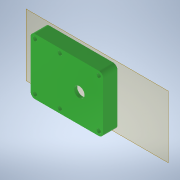
# Autodesk Inventor part: OutputFile
Saved by Autodesk Inventor 2022 (Build 260153000, 153)
## iProperties
Created: 2022-02-02
Part Number: OutputFile
Material: Generisch
Document SubType Name: Modeling
Designer: diederichbenedict
Density: 1 g/cm^3
Appearance: Glatt - Waldgrün
Mass: 24.3371 g
Surface Area: 140.293 cm^2
Volume: 24.3371 cm^3
Author: diederichbenedict
Autodesk Inventor part; units mm, degrees
ref_plane "YZ Plane" through (0, 0, 0) normal (1, 0, 0) x (0, 1, 0)
ref_plane "XZ Plane" through (0, 0, 0) normal (0, 1, 0) x (-1, 0, 0)
ref_plane "Arbeitsebene1" through (0, 0, 0) normal (0, 0, 1) x (1, 0, 0)
sketch "Skizze1" plane through (0, 0, 0) normal (0, 0, 1) x (1, 0, 0)
  arc A0 (-16.0148, -15.7672) -> (-14.255, -16.2126) centre (-14.255, -12.5126) ccw projected
  line L0 (-17.955, -12.5126) -> (-17.955, 12.4874) projected
  arc A1 (-14.255, 16.1874) -> (-17.955, 12.4874) centre (-14.255, 12.4874) ccw projected
  line L1 (-14.255, 16.1874) -> (23.745, 16.1874) projected
  arc A2 (25.6605, 15.6531) -> (23.745, 16.1874) centre (23.745, 12.4874) ccw projected
  arc A3 (26.3244, -15.1653) -> (27.445, -12.5126) centre (23.745, -12.5126) ccw projected
  line L2 (23.745, -16.2126) -> (-14.255, -16.2126) projected
  line L3 (-17.2153, 19.4874) -> (26.7847, 19.4874) projected
  arc A4 (-17.2153, 19.4874) -> (-20.2153, 16.4874) centre (-17.2153, 16.4874) ccw projected
  line L4 (-20.2153, -16.4874) -> (-20.2153, 16.4874) projected
  arc A5 (-20.2153, -16.4874) -> (-17.2153, -19.4874) centre (-17.2153, -16.4874) ccw projected
  line L5 (26.7847, -19.4874) -> (-17.2153, -19.4874) projected
  arc A6 (-16.0148, -15.7672) -> (-14.255, -16.2126) centre (-14.255, -12.5126) ccw projected
  line L6 (-17.955, -12.5126) -> (-17.955, 12.4874) projected
  arc A7 (-14.255, 16.1874) -> (-17.955, 12.4874) centre (-14.255, 12.4874) ccw projected
  line L7 (-14.255, 16.1874) -> (23.745, 16.1874) projected
  arc A8 (25.6605, 15.6531) -> (23.745, 16.1874) centre (23.745, 12.4874) ccw projected
  arc A9 (26.3244, -15.1653) -> (27.445, -12.5126) centre (23.745, -12.5126) ccw projected
  line L8 (23.745, -16.2126) -> (-14.255, -16.2126) projected
  line L9 (-17.2153, 19.4874) -> (26.7847, 19.4874) projected
  line L10 (26.7847, -19.4874) -> (-17.2153, -19.4874) projected
  line L11 (-20.2153, -16.4874) -> (-20.2153, 16.4874) projected
  arc A10 (-20.2153, -16.4874) -> (-17.2153, -19.4874) centre (-17.2153, -16.4874) ccw projected
  line L12 (29.7847, 16.4874) -> (29.7847, 15.1761) projected
  arc A11 (29.7847, 16.4874) -> (26.7847, 19.4874) centre (26.7847, 16.4874) ccw projected
  arc A12 (26.7847, -19.4874) -> (29.7847, -16.4874) centre (26.7847, -16.4874) ccw projected
  line L13 (29.7847, 16.4874) -> (29.7847, 15.1761) projected
  arc A13 (29.7847, 16.4874) -> (26.7847, 19.4874) centre (26.7847, 16.4874) ccw projected
  arc A14 (26.7847, -19.4874) -> (29.7847, -16.4874) centre (26.7847, -16.4874) ccw projected
  line L14 (28.445, 12.4874) -> (28.445, -12.5126)
  arc A15 (26.2819, 15.1808) -> (25.6605, 15.6531) centre (26.7847, 16.4874) ccw projected
  arc A16 (23.745, -16.2126) -> (25.6293, -15.6968) centre (23.745, -12.5126) ccw projected
  arc A17 (25.6293, -15.6968) -> (26.3244, -15.1653) centre (26.7847, -16.4874) ccw projected
  arc A18 (-16.8692, -15.1309) -> (-16.0148, -15.7672) centre (-17.2153, -16.4874) ccw projected
  arc A19 (27.3804, 13.1761) -> (26.2819, 15.1808) centre (23.745, 12.4874) ccw projected
  line L15 (23.745, 13.4874) -> (-14.255, 13.4874) projected
  line L16 (-14.255, -13.5126) -> (23.745, -13.5126) projected
  line L17 (25.0985, -12.5126) -> (27.445, -12.5126) projected
  arc A20 (-17.955, -12.5126) -> (-16.8692, -15.1309) centre (-14.255, -12.5126) ccw projected
  arc A21 (26.2819, 15.1808) -> (25.6605, 15.6531) centre (26.7847, 16.4874) ccw projected
  arc A22 (23.745, -16.2126) -> (25.6293, -15.6968) centre (23.745, -12.5126) ccw projected
  arc A23 (25.6293, -15.6968) -> (26.3244, -15.1653) centre (26.7847, -16.4874) ccw projected
  arc A24 (-16.8692, -15.1309) -> (-16.0148, -15.7672) centre (-17.2153, -16.4874) ccw projected
  arc A25 (27.3804, 13.1761) -> (26.2819, 15.1808) centre (23.745, 12.4874) ccw projected
  line L18 (23.745, 13.4874) -> (-14.255, 13.4874) projected
  line L19 (-14.255, -13.5126) -> (23.745, -13.5126) projected
  line L20 (25.0985, -12.5126) -> (27.445, -12.5126) projected
  arc A26 (-17.955, -12.5126) -> (-16.8692, -15.1309) centre (-14.255, -12.5126) ccw projected
  circle A27 centre (-17.2153, 16.4874) radius 1.15
  circle A28 centre (26.7847, 16.4874) radius 1.4
  circle A29 centre (26.7847, -16.4874) radius 1.4
  circle A30 centre (-17.2153, -16.4874) radius 1.4
  circle A31 centre (-17.2153, 16.4874) radius 1.15 projected
  circle A32 centre (-17.2153, 16.4874) radius 1.15 projected
  line L21 (25.0985, -9.7969) -> (25.0985, -12.5126) projected
  line L22 (18.0985, 10.1761) -> (-2.8285, 10.1761) projected
  line L23 (-2.8285, 10.1761) -> (-2.8285, 13.1761) projected
  arc A33 (24.4701, 13.1761) -> (23.745, 13.4874) centre (23.745, 12.4874) ccw projected
  arc A34 (23.745, -13.5126) -> (24.7038, -12.7969) centre (23.745, -12.5126) ccw projected
  line L24 (24.7038, -12.7969) -> (-2.8285, -12.7969) projected
  line L25 (-2.8285, -12.7969) -> (-2.8285, -9.7969) projected
  line L26 (-2.8285, -9.7969) -> (25.0985, -9.7969) projected
  circle A35 centre (-17.2153, 16.4874) radius 1.15 projected
  circle A36 centre (-17.2153, 16.4874) radius 1.15 projected
  line L27 (25.0985, -9.7969) -> (25.0985, -12.5126) projected
  line L28 (18.0985, 10.1761) -> (-2.8285, 10.1761) projected
  line L29 (-2.8285, 10.1761) -> (-2.8285, 13.1761) projected
  arc A37 (24.4701, 13.1761) -> (23.745, 13.4874) centre (23.745, 12.4874) ccw projected
  arc A38 (23.745, -13.5126) -> (24.7038, -12.7969) centre (23.745, -12.5126) ccw projected
  line L30 (24.7038, -12.7969) -> (-2.8285, -12.7969) projected
  line L31 (-2.8285, -12.7969) -> (-2.8285, -9.7969) projected
  line L32 (-2.8285, -9.7969) -> (25.0985, -9.7969) projected
  line L33 (27.445, 12.4874) -> (27.445, -12.5126)
  arc A39 (27.7847, 13.1761) -> (29.7847, 15.1761) centre (27.7847, 15.1761) ccw projected
  arc A40 (-17.2153, 19.4874) -> (-20.2153, 16.4874) centre (-17.2153, 16.4874) ccw projected
  line L34 (29.7847, 2.2345) -> (29.7847, -16.4874) projected
  arc A41 (29.7847, 2.2345) -> (27.7847, 4.2345) centre (27.7847, 2.2345) ccw projected
  line L35 (27.7847, 4.2345) -> (22.0985, 4.2345) projected
  arc A42 (20.0985, 6.2345) -> (22.0985, 4.2345) centre (22.0985, 6.2345) ccw projected
  line L36 (20.0985, 6.2345) -> (20.0985, 8.1761) projected
  arc A43 (20.0985, 8.1761) -> (18.0985, 10.1761) centre (18.0985, 8.1761) ccw projected
  line L37 (-2.8285, 13.1761) -> (24.4701, 13.1761) projected
  arc A44 (-14.255, 13.4874) -> (-15.255, 12.4874) centre (-14.255, 12.4874) ccw projected
  line L38 (-15.255, 12.4874) -> (-15.255, -12.5126) projected
  arc A45 (-15.255, -12.5126) -> (-14.255, -13.5126) centre (-14.255, -12.5126) ccw projected
  line L39 (27.3804, 13.1761) -> (27.7847, 13.1761) projected
  arc A46 (27.7847, 13.1761) -> (29.7847, 15.1761) centre (27.7847, 15.1761) ccw projected
  line L40 (29.7847, 2.2345) -> (29.7847, -16.4874) projected
  arc A47 (29.7847, 2.2345) -> (27.7847, 4.2345) centre (27.7847, 2.2345) ccw projected
  line L41 (27.7847, 4.2345) -> (22.0985, 4.2345) projected
  arc A48 (20.0985, 6.2345) -> (22.0985, 4.2345) centre (22.0985, 6.2345) ccw projected
  line L42 (20.0985, 6.2345) -> (20.0985, 8.1761) projected
  arc A49 (20.0985, 8.1761) -> (18.0985, 10.1761) centre (18.0985, 8.1761) ccw projected
  line L43 (-2.8285, 13.1761) -> (24.4701, 13.1761) projected
  arc A50 (-14.255, 13.4874) -> (-15.255, 12.4874) centre (-14.255, 12.4874) ccw projected
  line L44 (-15.255, 12.4874) -> (-15.255, -12.5126) projected
  arc A51 (-15.255, -12.5126) -> (-14.255, -13.5126) centre (-14.255, -12.5126) ccw projected
  line L45 (27.3804, 13.1761) -> (27.7847, 13.1761) projected
  line L46 (27.3804, 13.1761) -> (27.445, 12.4874)
  line L47 (29.7847, 2.2345) -> (29.7847, 15.1761)
  point P0 (0, 0)
  point P1 (-15.255, 11.1874)
  point P2 (23.745, 12.4874)
  point P3 (23.745, -12.5126)
  point P4 (-17.8427, 15.5236)
  point P5 (-14.255, 12.4874)
  point P6 (-16.1103, 16.8058)
  point P7 (-14.255, 12.4874)
  point P8 (-17.2153, -19.4874)
  point P9 (25.0985, 12.4874)
  point P10 (25.0985, 10.1761)
  point P11 (27.445, -12.5126)
  point P12 (26.3244, -15.1653)
  point P13 (25.6293, -15.6968)
  point P14 (-16.0148, -15.7672)
  point P15 (-16.8692, -15.1309)
  point P16 (25.6605, 15.6531)
  point P17 (26.2819, 15.1808)
  point P18 (29.7847, 15.1761)
  point P19 (25.6605, 15.6531)
  point P20 (26.2819, 15.1808)
  point P21 (27.445, 4.2345)
  constraints: 8 end point, 4 coincident, 3 centre point, 3 concentric, 2 point on circle, 2 vertical, 1 parallel, 4 other
ref_plane "Arbeitsebene2" through (-3.9015, -6.25, 7.6898) normal (0, 0, 1) x (1, 0, 0)
extrude "Extrusion1" add sketch "Skizze1" along normal up to surface (7.6898 mm away) contours A0 L2 A16 A17 A3 L33 L35 A41 L34 A12 L5 A5 L4 A4 L3 A11 L12 A39 L39 A19 A15 A2 L1 A1 L0 A20 A18 | L33 L46 L39 A39 L47 A41 L35
sketch "Skizze2" plane through (-17.2153, -19.4874, 7.6898) normal (0, 0, 1) x (1, 0, 0)
  arc A0 (0, 38.9749) -> (-3, 35.9749) centre (0, 35.9749) ccw
  line L0 (-3, 3) -> (-3, 35.9749)
  arc A1 (-3, 3) -> (0, 0) centre (0, 3) ccw
  circle A2 centre (30.5638, 19.4874) radius 3.6158
  arc A3 (44, 0) -> (47, 3) centre (44, 3) ccw
  arc A4 (47, 35.9749) -> (44, 38.9749) centre (44, 35.9749) ccw
  line L1 (0, 38.9749) -> (44, 38.9749)
  line L2 (44, 0) -> (0, 0)
  circle A5 centre (30.5638, 19.4874) radius 3.6158
  line L3 (34.6638, 15.3874) -> (26.4638, 15.3874)
  line L4 (26.4638, 15.3874) -> (26.4638, 23.5874)
  line L5 (26.4638, 23.5874) -> (34.6638, 23.5874)
  line L6 (34.6638, 23.5874) -> (34.6638, 15.3874)
  line L7 (34.6638, 15.3874) -> (26.4638, 23.5874) construction
  line L8 (26.4638, 15.3874) -> (34.6638, 23.5874) construction
  arc A6 (0.3462, 4.3565) -> (1.2005, 3.7202) centre (0, 3) ccw
  circle A7 centre (0, 35.9749) radius 1.15
  arc A8 (43.4972, 34.6683) -> (42.8758, 35.1405) centre (44, 35.9749) ccw
  arc A9 (42.8446, 3.7906) -> (43.5397, 4.3222) centre (44, 3) ccw
  arc A10 (-3, 3) -> (0, 0) centre (0, 3) ccw
  circle A11 centre (0, 3) radius 1.4
  circle A12 centre (0, 35.9749) radius 1.4
  circle A13 centre (44, 35.9749) radius 1.4
  circle A14 centre (44, 3) radius 1.4
  circle A15 centre (30.5638, 19.4874) radius 3.75
  line L9 (44.6604, 6.9749) -> (44.6604, 31.9749)
  arc A16 (43.5397, 4.3222) -> (44.6604, 6.9749) centre (40.9604, 6.9749) ccw
  arc A17 (42.8446, 3.7906) -> (43.5397, 4.3222) centre (44, 3) ccw
  arc A18 (40.9604, 3.2749) -> (42.8446, 3.7906) centre (40.9604, 6.9749) ccw
  line L10 (2.9604, 3.2749) -> (40.9604, 3.2749)
  arc A19 (1.2005, 3.7202) -> (2.9604, 3.2749) centre (2.9604, 6.9749) ccw
  arc A20 (0.3462, 4.3565) -> (1.2005, 3.7202) centre (0, 3) ccw
  arc A21 (-0.7396, 6.9749) -> (0.3462, 4.3565) centre (2.9604, 6.9749) ccw
  line L11 (-0.7396, 31.9749) -> (-0.7396, 6.9749)
  arc A22 (2.9604, 35.6749) -> (-0.7396, 31.9749) centre (2.9604, 31.9749) ccw
  line L12 (40.9604, 35.6749) -> (2.9604, 35.6749)
  arc A23 (42.8758, 35.1405) -> (40.9604, 35.6749) centre (40.9604, 31.9749) ccw
  arc A24 (43.4972, 34.6683) -> (42.8758, 35.1405) centre (44, 35.9749) ccw
  arc A25 (44.5957, 32.6636) -> (43.4972, 34.6683) centre (40.9604, 31.9749) ccw
  line L13 (47, 35.9749) -> (47, 3)
  line L14 (44.6604, 31.9749) -> (44.5957, 32.6636)
  point P0 (17.2153, 19.4874)
  point P1 (0.3462, 4.3565)
  point P2 (1.2005, 3.7202)
  point P3 (43.4972, 34.6683)
  point P4 (42.8758, 35.1405)
  point P5 (42.8446, 3.7906)
  point P6 (43.5397, 4.3222)
extrude "Extrusion2" add sketch "Skizze2" along normal blind 2.2 contours L1 A4 L13 A3 L2 A1 L0 A0 | L3 L4 L5 L6 | A11 A6 | A21 L11 A22 A12 L12 A23 A13 A25 L14 L9 A16 A14 A18 L10 A19 A11 | A22 A12 | A12 A22 | A14 A9 | A8 A13 | A15
sketch "Sketch13" plane through (-17.2153, -19.4874, 9.8898) normal (0, 0, 1) x (1, 0, 0)
  circle A0 centre (30.5638, 19.4874) radius 7 projected
  circle A1 centre (44, 3) radius 1.4 projected
  circle A2 centre (44, 35.9749) radius 1.4 projected
  line L0 (17.1276, 35.9749) -> (44, 35.9749)
  line L1 (44, 35.9749) -> (44, 3)
  line L2 (44, 3) -> (17.1276, 3)
  line L3 (17.1276, 3) -> (17.1276, 35.9749)
  line L4 (17.1276, 35.9749) -> (44, 3) construction
  line L5 (44, 35.9749) -> (17.1276, 3) construction
  circle A3 centre (0, 35.9749) radius 1.15 projected
  circle A4 centre (0, 3) radius 1.4 projected
  point P0 (17.2153, 19.4874)
  constraints: 12 end point, 2 midpoint, 2 parallel, 1 horizontal, 1 perpendicular
hole "Hole1" at (26.7847, -16.4874, 9.8898) at (-0.0877, -16.4874, 9.8898) at (-0.0877, 16.4874, 9.8898) at (26.7847, 16.4874, 9.8898) at (-17.2153, 16.4874, 9.8898) at (-17.2153, -16.4874, 9.8898) direction (0, 0, -1) diameter 2.9 depth 15 tip angle 118
equation "\"d50\" = 0.125 * Sketch7_Pitch"
equation "\"Sketch7_Pitch\" = 1"
equation "\"d52\" = 60deg"
